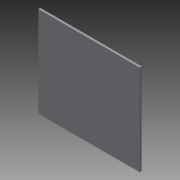
# Autodesk Inventor part: Plate
Saved by Autodesk Inventor 2014 (Build 180170000, 170)
## iProperties
Created: 2014-01-05
Part Number: Plate
Material: Generic
Document SubType Name: Modeling
Designer: Tristan Debrunner
Density: 1 g/cm^3
Appearance: Default
Author: Tristan Debrunner
Autodesk Inventor part; units mm, degrees
ref_plane "YZ Plane" through (0, 0, 0) normal (1, 0, 0) x (0, 1, 0)
ref_plane "XZ Plane" through (0, 0, 0) normal (0, 1, 0) x (-1, 0, 0)
ref_plane "XY Plane" through (0, 0, 0) normal (0, 0, 1) x (1, 0, 0)
sketch "Sketch1" plane through (0, 0, 0) normal (0, 0, 1) x (1, 0, 0)
  line L0 (-624.9675, 558.4224) -> (624.9675, 558.4224)
  line L1 (624.9675, 558.4224) -> (624.9675, -558.4224)
  line L2 (624.9675, -558.4224) -> (-624.9675, -558.4224)
  line L3 (-624.9675, -558.4224) -> (-624.9675, 558.4224)
  line L4 (-624.9675, 558.4224) -> (624.9675, -558.4224) construction
  line L5 (624.9675, 558.4224) -> (-624.9675, -558.4224) construction
  point P0 (0, 0)
  constraints: 12 end point, 2 midpoint, 2 parallel, 1 horizontal, 1 perpendicular
extrude "Extrusion1" add sketch "Sketch1" along normal blind 25.4
body "Solid1"
